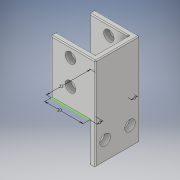
# Autodesk Inventor part: bottom printhead screwplate_250221
Saved by Autodesk Inventor 2019 (Build 230136000, 136)
## iProperties
Created: 2021-02-20
Part Number: bottom printhead screwplate_250221
Material: Generic
Document SubType Name: Modeling
Designer: Iek Man Lei
Density: 1 g/cm^3
Appearance: Default
Author: Iek Man Lei
Autodesk Inventor part; units mm, degrees
ref_plane "YZ Plane" through (0, 0, 0) normal (1, 0, 0) x (0, 1, 0)
ref_plane "XZ Plane" through (0, 0, 0) normal (0, 1, 0) x (-1, 0, 0)
ref_plane "XY Plane" through (0, 0, 0) normal (0, 0, 1) x (1, 0, 0)
sketch "Sketch1" plane through (0, 0, 0) normal (0, 1, 0) x (-1, 0, 0)
  line L0 (7.8238, 10.3217) -> (-12.1762, 10.3217)
  line L1 (-12.1762, 10.3217) -> (-12.1762, -12.6783)
  line L2 (-12.1762, -12.6783) -> (7.8238, -12.6783)
  line L3 (7.8238, -12.6783) -> (7.8238, 10.3217)
  line L4 (7.8238, 10.3217) -> (-12.1762, 10.3217)
  line L5 (-12.1762, 10.3217) -> (-12.1762, 7.3217)
  line L6 (-12.1762, 7.3217) -> (7.8238, 7.3217)
  line L7 (7.8238, 7.3217) -> (7.8238, 10.3217)
  line L8 (7.8238, -12.6783) -> (-12.1762, -12.6783)
  line L9 (-12.1762, -12.6783) -> (-12.1762, -9.6783)
  line L10 (-12.1762, -9.6783) -> (7.8238, -9.6783)
  line L11 (7.8238, -9.6783) -> (7.8238, -12.6783)
  point P0 (0, 0)
  dimension "d0" = 23
  dimension "d1" = 20
  dimension "d2" = 3
  dimension "d3" = 3
  constraints: 24 end point, 6 parallel, 3 horizontal, 3 perpendicular, 2 point on line
  measures "d0" distance of L2.end L0.start
  measures "d1" distance of L0.start L0.end
  measures "d2" distance of L1.end L9.end
  measures "d3" distance of L0.end L5.end
extrude "Extrusion1" add sketch "Sketch1" along normal blind 28 contours L3 L6 L1 L0 | L3 L2 L1 L10
sketch "Sketch2" plane through (-7.8238, 0, 10.3217) normal (0, 0, 1) x (1, 0, 0)
  circle A0 centre (10, 10) radius 2.75
  circle A1 centre (10, 23) radius 2.75
  line L0 (0, 0) -> (20, 0) projected
  line L1 (0, 28) -> (20, 28) projected
  line L2 (0, 0) -> (0, 28) projected
  point P0 (7.8238, 0)
  dimension "d6" = 5.5
  dimension "d7" = 5.5
  dimension "d8" = 10
  dimension "d9" = 5
  dimension "d10" = 10
  constraints: 2 centre point, 1 vertical alignment
  measures "d6" diameter of A0
  measures "d7" diameter of A1
  measures "d8" distance from line of L0 A0.centre
  measures "d9" distance from line of A1.centre L1
  measures "d10" distance from line of A0.centre L2
extrude "Extrusion2" cut sketch "Sketch2" against normal through all
sketch "Sketch3" plane through (12.1762, 0, -9.6783) normal (1, 0, 0) x (0, 0, -1)
  line L0 (3, 28) -> (-20, 28)
  line L1 (-20, 28) -> (-20, -20)
  line L2 (-20, -20) -> (3, -20)
  line L3 (3, -20) -> (3, 28)
  point P0 (-9.6783, 0)
  dimension "d13" = 48
  constraints: 8 end point, 2 parallel, 1 coincident, 1 horizontal, 1 perpendicular
  measures "d13" distance of L2.end L0.start
extrude "Extrusion3" add sketch "Sketch3" along normal blind 3
sketch "Sketch4" plane through (15.1762, 0, -9.6783) normal (1, 0, 0) x (0, 0, -1)
  circle A0 centre (-15, -10) radius 2.75
  line L0 (-20, -20) -> (3, -20) projected
  line L1 (-20, 28) -> (-20, -20) projected
  circle A1 centre (-2, -10) radius 2.75
  line L2 (3, -20) -> (3, 28) projected
  point P0 (-9.6783, 0)
  dimension "d16" = 5.5
  dimension "d17" = 10
  dimension "d18" = 5
  dimension "d21" = 13
  dimension "d26" = 5
  constraints: 2 centre point, 1 horizontal, 2 other
  measures "d16" diameter of A0
  measures "d17" distance from line of A0.centre L0
  measures "d18" distance from line of L1 A0.centre
  measures "d21" distance of A0.centre A1.centre
  measures "d26" distance from line of L2 A1.centre
extrude "Extrusion4" cut sketch "Sketch4" against normal blind 3
fillet "Fillet1" radius 0.5 3 edges at (12.1762, -10, 10.3217) (15.1762, 4, 10.3217) (-7.8238, 14, 10.3217)
fillet "Fillet1" radius 0.5 17 edges at (-7.8238, 14, 7.3217) (-7.8238, 14, -9.6783) (-7.8238, 14, -12.6783) (2.1762, 28, 7.3217) (12.1762, 28, -1.1783) (2.1762, 28, -9.6783) (3.6762, 28, -12.6783) (15.1762, 28, -1.1783) (3.6762, 28, 10.3217) (12.1762, -10, -12.6783) (15.1762, 4, -12.6783) (12.1762, -20, -1.1783) (15.1762, -20, -1.1783) (2.1762, 0, 7.3217) (2.1762, 0, 10.3217) (2.1762, 0, -9.6783) (2.1762, 0, -12.6783)
fillet "Fillet2" radius 0.5 10 edges at (12.3227, 27.8536, 7.4682) (12.1762, 0.1464, 7.4682) (12.1762, 0, 8.8217) (12.3227, 0.1464, 10.1753) (12.1762, 14, 7.3217) (12.3227, 27.8536, -9.8247) (12.1762, 0.1464, -9.8247) (12.1762, 0, -11.1783) (12.3227, 0.1464, -12.5318) (12.1762, 14, -9.6783)
body "Solid1"
